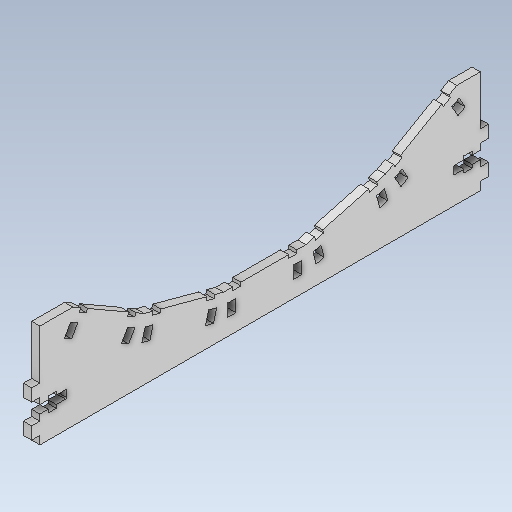
# Autodesk Inventor part: switchplate-support-04
Saved by Autodesk Inventor 2020.1 (Build 241239000, 239)
## iProperties
Created: 2019-06-27
Material: Acier, galvanisé
Document SubType Name: Modeling
Designer: Thibault
Density: 7.85 g/cm^3
Appearance: Anodisé - Bronze foncé subtil
Mass: 11.7255 g
Surface Area: 33.7109 cm^2
Volume: 1.4937 cm^3
Part Number: switchplate-support-04
sa_0: 0.400 nd
height_shift: 0,000 mm
base_height: 25,000 mm
switchplate_depth: 111,000 mm
Author: Thibault
Autodesk Inventor part; units mm, degrees
ref_plane "YZ Plane" through (0, 0, 0) normal (1, 0, 0) x (0, 1, 0)
ref_plane "XZ Plane" through (0, 0, 0) normal (0, 1, 0) x (-1, 0, 0)
ref_plane "XY Plane" through (0, 0, 0) normal (0, 0, 1) x (1, 0, 0)
sketch "Anchor (screw side)" plane through (0, 0, 0) normal (0, 0, 1) x (1, 0, 0)
  circle A0 centre (93.7814, 50.2592) radius 1
  line L0 (91.2814, 51.2592) -> (88.2814, 51.2592)
  line L1 (88.2814, 51.2592) -> (88.2814, 49.2592)
  line L2 (88.2814, 49.2592) -> (91.2814, 49.2592)
  line L3 (91.2814, 49.2592) -> (91.2814, 51.2592)
  line L4 (99.2814, 51.2592) -> (96.2814, 51.2592)
  line L5 (96.2814, 51.2592) -> (96.2814, 49.2592)
  line L6 (96.2814, 49.2592) -> (99.2814, 49.2592)
  line L7 (99.2814, 49.2592) -> (99.2814, 51.2592)
  line L8 (91.2814, 51.2592) -> (96.2814, 49.2592) construction
  line L9 (96.2814, 51.2592) -> (91.2814, 49.2592) construction
  line L10 (86.2814, 53.2592) -> (101.2814, 53.2592) construction
  line L11 (101.2814, 53.2592) -> (101.2814, 47.2592) construction
  line L12 (101.2814, 47.2592) -> (86.2814, 47.2592) construction
  line L13 (86.2814, 47.2592) -> (86.2814, 53.2592) construction
  point P0 (103.5798, 50.1132)
  dimension "d27_1" = 2
  dimension "d28_1" = 3
  dimension "d29" = 2
  dimension "d30" = 3
  dimension "d32" = 5
  dimension "d34" = 2
  dimension "d35" = 2
  dimension "d36" = 2
  dimension "d37" = 2
  measures "d27_1" diameter of A0
  measures "d28_1" distance of L2.end L1.end
  measures "d29" distance of L1.end L0.end
  measures "d30" distance of L6.end L5.end
  measures "d32" distance between parallel lines of L5 L3
  measures "d34" distance between parallel lines of L0 L10
  measures "d35" distance between parallel lines of L12 L2
  measures "d36" distance between parallel lines of L11 L7
  measures "d37" distance between parallel lines of L13 L1
sketch "Anchor (nut side)" plane through (0, 0, 0) normal (0, 0, 1) x (1, 0, 0)
  line L0 (10, 0) -> (8.5, 0)
  line L1 (8.5, 0) -> (8.5, -2)
  line L2 (8.5, -2) -> (9.3, -2)
  line L3 (9.3, -2) -> (9.3, -4)
  line L4 (5.7, -4) -> (5.7, -2)
  line L5 (5.7, -2) -> (6.5, -2)
  line L6 (6.5, -2) -> (6.5, 0)
  line L7 (6.5, 0) -> (5, 0)
  line L8 (2, 0) -> (2, 2)
  line L9 (2, 0) -> (3, 0) construction
  line L10 (2, 2) -> (5, 2)
  line L11 (5, 2) -> (5, 0)
  line L12 (5, 2) -> (7, 2) construction
  line L13 (10, 0) -> (10, 2)
  line L14 (10, 2) -> (13, 2)
  line L15 (13, 2) -> (13, 0)
  line L16 (0, 0) -> (2, 0)
  line L17 (13, 0) -> (15, 0)
  line L18 (5.7, -4) -> (6.5, -4)
  line L19 (9.3, -4) -> (8.5, -4)
  line L20 (6.5, -4) -> (6.5, -6.25)
  line L21 (8.5, -4) -> (8.5, -6.25)
  line L22 (6.75, -6.5) -> (7.5, -6.5)
  arc A0 (6.5, -6.25) -> (6.75, -6.5) centre (6.75, -6.25) ccw
  arc A1 (8.25, -6.5) -> (8.5, -6.25) centre (8.25, -6.25) ccw
  line L23 (7.5, -7.2938) -> (7.5, -4.9797)
  line L24 (7.5, -6.5) -> (8.25, -6.5)
  point P0 (9.1321, -0.6227)
  point P1 (6.5, -6.5)
  point P2 (8.5, -6.5)
  dimension "d3" = 2
  dimension "d7" = 5
  dimension "d10" = 1.5
  dimension "d11" = 2
  dimension "d12" = 0.8
  dimension "d13" = 2
  dimension "d14" = 0.8
  dimension "d15" = 2
  dimension "d18" = 2
  dimension "d19" = 0.8
  dimension "d20" = 0.8
  dimension "d21" = 2.5
  dimension "d22" = 2.5
  dimension "d23" = 2
  dimension "d38" = 2
  dimension "d39" = 0.25
  dimension "d118" = 2
  dimension "d120" = 3
  measures "d3" distance of point (0, 0) L8.start
  measures "d7" distance of L7.end L0.start
  measures "d10" distance of L0.start L0.end
  measures "d11" distance of L0.end L1.end
  measures "d12" distance of L1.end L2.end
  measures "d13" distance of L2.end L3.end
  measures "d14" distance of L4.end L5.end
  measures "d15" distance of L6.end L0.end
  measures "d18" distance of L15.end point (15, 0)
  measures "d19" distance of L4.start L18.end
  measures "d20" distance of L3.end L19.end
  measures "d21" distance of L18.end point (6.5, -6.5)
  measures "d22" distance of L19.end point (8.5, -6.5)
  measures "d23" distance of L18.end L19.end
  measures "d38" distance of the line from the sketch origin of L10
  measures "d39" radius of A0
  measures "d118" distance between parallel lines of L0 L14
  measures "d120" distance of L8.end L10.end
sketch "Anchor (to 2ndary key support)" plane through (0, 0, 0) normal (0, 0, 1) x (1, 0, 0)
  line L0 (12.7767, 14.8837) -> (14.7767, 14.8837)
  line L1 (14.7767, 14.8837) -> (14.7767, 11.8837)
  line L2 (14.7767, 11.8837) -> (12.7767, 11.8837)
  line L3 (12.7767, 11.8837) -> (12.7767, 14.8837)
  point P0 (14.0267, 11.8837)
  dimension "d40" = 2
  dimension "d41" = 3
  measures "d40" distance of L1.end L2.end
  measures "d41" distance of L0.end L1.end
sketch "Switch support" plane through (0, 0, 0) normal (0, 0, 1) x (1, 0, 0)
  line L0 (14.375, 16.4474) -> (15.075, 16.4474)
  line L1 (15.075, 16.4474) -> (15.075, 15.6474)
  line L2 (15.075, 15.6474) -> (17.075, 15.6474)
  line L3 (17.075, 15.6474) -> (17.075, 16.4474)
  line L4 (17.075, 16.4474) -> (22.875, 16.4474)
  line L5 (28.675, 16.4474) -> (28.675, 15.6474)
  line L6 (28.675, 15.6474) -> (30.675, 15.6474)
  line L7 (30.675, 15.6474) -> (30.675, 16.4474)
  line L8 (30.675, 16.4474) -> (31.375, 16.4474)
  line L9 (22.875, 19.1721) -> (22.875, 15.8971) construction
  line L10 (22.875, 16.4474) -> (28.675, 16.4474)
  line L11 (13.875, 13.6474) -> (15.875, 13.6474)
  line L12 (15.875, 13.6474) -> (15.875, 10.6474)
  line L13 (15.875, 10.6474) -> (13.875, 10.6474)
  line L14 (13.875, 10.6474) -> (13.875, 13.6474)
  line L15 (29.875, 13.6474) -> (31.875, 13.6474)
  line L16 (31.875, 13.6474) -> (31.875, 10.6474)
  line L17 (31.875, 10.6474) -> (29.875, 10.6474)
  line L18 (29.875, 10.6474) -> (29.875, 13.6474)
  point P0 (20.0288, 26.7181)
  dimension "d43" = 0.8
  dimension "d44" = 2
  dimension "d45" = 11.6
  dimension "d46" = 2
  dimension "d47" = 0.7
  dimension "d48" = 17
  dimension "d49" = 7
  dimension "d50" = 7
  dimension "d51" = 2
  measures "d43" distance of L1.start L1.end
  measures "d44" distance of L1.end L2.end
  measures "d45" distance of L5.start L3.end
  measures "d46" distance of L5.end L6.end
  measures "d47" distance of L7.end point (31.375, 16.447)
  measures "d48" distance of point (31.375, 16.447) point (14.375, 16.447)
  measures "d51" length of L2
sketch "Sketch1" plane through (0, 0, 0) normal (1, 0, 0) x (0, 1, 0)
  line L0 (0, -111) -> (25, -111)
  line L1 (0, 0) -> (0, -111)
  line L2 (25, 0) -> (0, 0)
  line L3 (25, -111) -> (25, -103.278)
  line L4 (24.4162, -11.0111) -> (25, -10)
  line L5 (28.2121, -16.9724) -> (22.1003, -16.9724)
  line L6 (24.25, -11.299) -> (25, -10)
  line L7 (15.75, -26.0215) -> (15, -27.3205)
  line L8 (21.9473, -35.6102) -> (15.8356, -35.6102)
  line L9 (14.6118, -28.7694) -> (15, -27.3205)
  line L10 (10.2118, -45.1901) -> (9.8236, -46.639)
  line L11 (19.8511, -55.1756) -> (13.7394, -55.1756)
  line L12 (9.8236, -48.139) -> (9.8236, -46.639)
  line L13 (9.8236, -65.139) -> (9.8236, -66.639)
  line L14 (22.0358, -74.7409) -> (15.9241, -74.7409)
  line L15 (10.2118, -68.0879) -> (9.8236, -66.639)
  line L16 (14.6118, -84.5087) -> (15, -85.9575)
  line L17 (28.3566, -93.3787) -> (22.2449, -93.3787)
  line L18 (15.75, -87.2566) -> (15, -85.9575)
  line L19 (24.25, -101.979) -> (25, -103.278)
  line L20 (25, 0) -> (25, -10)
  line L21 (14.6118, -28.7694) -> (14.4306, -29.4455)
  line L22 (14.4306, -29.4455) -> (13.6579, -29.2385)
  line L23 (13.6579, -29.2385) -> (13.1402, -31.1703)
  line L24 (13.1402, -31.1703) -> (13.913, -31.3774)
  line L25 (13.913, -31.3774) -> (12.4118, -36.9798)
  line L26 (10.9107, -42.5821) -> (10.1379, -42.3751)
  line L27 (10.1379, -42.3751) -> (9.6203, -44.3069)
  line L28 (9.6203, -44.3069) -> (10.393, -44.514)
  line L29 (10.393, -44.514) -> (10.2118, -45.1901)
  line L30 (15.0436, -37.685) -> (11.8802, -36.8373) construction
  line L31 (12.4118, -36.9798) -> (10.9107, -42.5821)
  line L32 (12.0366, -27.5617) -> (11.519, -29.4936)
  line L33 (11.519, -29.4936) -> (8.6212, -28.7171)
  line L34 (8.6212, -28.7171) -> (9.1388, -26.7853)
  line L35 (9.1388, -26.7853) -> (12.0366, -27.5617)
  line L36 (7.8955, -43.0166) -> (7.3778, -44.9484)
  line L37 (7.3778, -44.9484) -> (4.4801, -44.1719)
  line L38 (4.4801, -44.1719) -> (4.9977, -42.2401)
  line L39 (4.9977, -42.2401) -> (7.8955, -43.0166)
  line L40 (24.25, -11.299) -> (23.9, -11.9053)
  line L41 (23.9, -11.9053) -> (23.2072, -11.5053)
  line L42 (23.2072, -11.5053) -> (22.2072, -13.2373)
  line L43 (22.2072, -13.2373) -> (22.9, -13.6373)
  line L44 (22.9, -13.6373) -> (20, -18.6603)
  line L45 (17.1, -23.6832) -> (16.4072, -23.2832)
  line L46 (16.4072, -23.2832) -> (15.4072, -25.0153)
  line L47 (15.4072, -25.0153) -> (16.1, -25.4153)
  line L48 (16.1, -25.4153) -> (15.75, -26.0215)
  line L49 (22.3596, -20.0226) -> (19.5234, -18.3851) construction
  line L50 (20, -18.6603) -> (17.1, -23.6832)
  line L51 (22.0751, -9.466) -> (21.0751, -11.1981)
  line L52 (21.0751, -11.1981) -> (18.4771, -9.6981)
  line L53 (18.4771, -9.6981) -> (19.4771, -7.966)
  line L54 (19.4771, -7.966) -> (22.0751, -9.466)
  line L55 (14.0751, -23.3224) -> (13.0751, -25.0545)
  line L56 (13.0751, -25.0545) -> (10.4771, -23.5545)
  line L57 (10.4771, -23.5545) -> (11.4771, -21.8224)
  line L58 (11.4771, -21.8224) -> (14.0751, -23.3224)
  line L59 (9.8236, -48.139) -> (9.8236, -48.839)
  line L60 (9.8236, -48.839) -> (9.0236, -48.839)
  line L61 (9.0236, -48.839) -> (9.0236, -50.839)
  line L62 (9.0236, -50.839) -> (9.8236, -50.839)
  line L63 (9.8236, -50.839) -> (9.8236, -56.639)
  line L64 (9.8236, -62.439) -> (9.0236, -62.439)
  line L65 (9.0236, -62.439) -> (9.0236, -64.439)
  line L66 (9.0236, -64.439) -> (9.8236, -64.439)
  line L67 (9.8236, -64.439) -> (9.8236, -65.139)
  line L68 (12.5483, -56.639) -> (9.2733, -56.639) construction
  line L69 (9.8236, -56.639) -> (9.8236, -62.439)
  line L70 (7.0236, -47.639) -> (7.0236, -49.639)
  line L71 (7.0236, -49.639) -> (4.0236, -49.639)
  line L72 (4.0236, -49.639) -> (4.0236, -47.639)
  line L73 (4.0236, -47.639) -> (7.0236, -47.639)
  line L74 (7.0236, -63.639) -> (7.0236, -65.639)
  line L75 (7.0236, -65.639) -> (4.0236, -65.639)
  line L76 (4.0236, -65.639) -> (4.0236, -63.639)
  line L77 (4.0236, -63.639) -> (7.0236, -63.639)
  line L78 (10.2118, -68.0879) -> (10.393, -68.7641)
  line L79 (10.393, -68.7641) -> (9.6203, -68.9711)
  line L80 (9.6203, -68.9711) -> (10.1379, -70.903)
  line L81 (10.1379, -70.903) -> (10.9107, -70.6959)
  line L82 (10.9107, -70.6959) -> (12.4118, -76.2983)
  line L83 (13.913, -81.9007) -> (13.1402, -82.1077)
  line L84 (13.1402, -82.1077) -> (13.6579, -84.0396)
  line L85 (13.6579, -84.0396) -> (14.4306, -83.8325)
  line L86 (14.4306, -83.8325) -> (14.6118, -84.5087)
  line L87 (15.0436, -75.5931) -> (11.8802, -76.4407) construction
  line L88 (12.4118, -76.2983) -> (13.913, -81.9007)
  line L89 (7.3778, -68.3296) -> (7.8955, -70.2615)
  line L90 (7.8955, -70.2615) -> (4.9977, -71.038)
  line L91 (4.9977, -71.038) -> (4.4801, -69.1061)
  line L92 (4.4801, -69.1061) -> (7.3778, -68.3296)
  line L93 (11.519, -83.7845) -> (12.0366, -85.7163)
  line L94 (12.0366, -85.7163) -> (9.1388, -86.4928)
  line L95 (9.1388, -86.4928) -> (8.6212, -84.5609)
  line L96 (8.6212, -84.5609) -> (11.519, -83.7845)
  line L97 (15.75, -87.2566) -> (16.1, -87.8628)
  line L98 (16.1, -87.8628) -> (15.4072, -88.2628)
  line L99 (15.4072, -88.2628) -> (16.4072, -89.9948)
  line L100 (16.4072, -89.9948) -> (17.1, -89.5948)
  line L101 (17.1, -89.5948) -> (20, -94.6178)
  line L102 (22.9, -99.6407) -> (22.2072, -100.0407)
  line L103 (22.2072, -100.0407) -> (23.2072, -101.7728)
  line L104 (23.2072, -101.7728) -> (23.9, -101.3728)
  line L105 (23.9, -101.3728) -> (24.25, -101.979)
  line L106 (22.3596, -93.2555) -> (19.5234, -94.893) construction
  line L107 (20, -94.6178) -> (22.9, -99.6407)
  line L108 (13.0751, -88.2236) -> (14.0751, -89.9556)
  line L109 (14.0751, -89.9556) -> (11.4771, -91.4556)
  line L110 (11.4771, -91.4556) -> (10.4771, -89.7236)
  line L111 (10.4771, -89.7236) -> (13.0751, -88.2236)
  line L112 (21.0751, -102.08) -> (22.0751, -103.812)
  line L113 (22.0751, -103.812) -> (19.4771, -105.312)
  line L114 (19.4771, -105.312) -> (18.4771, -103.58)
  line L115 (18.4771, -103.58) -> (21.0751, -102.08)
  point P0 (24.25, -101.979)
  point P1 (15.75, -87.2566)
  point P2 (14.6118, -84.5087)
  point P3 (10.2118, -68.0879)
  point P4 (9.8236, -65.139)
  point P5 (9.8236, -48.139)
  point P6 (10.2118, -45.1901)
  point P7 (14.6118, -28.7694)
  point P8 (15.75, -26.0215)
  dimension "height" = 25
  dimension "d193" = 25
  dimension "k1_a" = 1.5
  dimension "k1_b" = 1.5
  dimension "k2_a" = 1.5
  dimension "k2_b" = 1.5
  dimension "k3_a" = 1.5
  dimension "k3_b" = 1.5
  dimension "k4_a" = 1.5
  dimension "k4_b" = 1.5
  dimension "k5_a" = 1.5
  dimension "k5_b" = 1.5
  dimension "d257" = 10
  dimension "k1_angle" = 120
  dimension "k2_angle" = 105
  dimension "k3_angle" = 90
  dimension "k4_angle" = 75
  dimension "k5_angle" = 60
  constraints: 42 end point, 7 horizontal, 4 vertical, 1 collinear, 1 vertical alignment, 19 other
  measures "height" distance of L2.start L1.start
  measures "d193" distance of L0.end L0.start
  measures "k1_a" distance of L4.end L6.start
  measures "k1_b" distance of L7.end L7.start
  measures "k2_a" distance of L9.start L7.end
  measures "k2_b" distance of L10.end L10.start
  measures "k3_a" distance of L12.start L10.end
  measures "k3_b" distance of L13.end L13.start
  measures "k4_a" distance of L15.start L13.end
  measures "k4_b" distance of L16.end L16.start
  measures "k5_a" distance of L18.start L16.end
  measures "k5_b" distance of L3.end L19.start
  measures "d257" distance of L2.start L4.end
  measures "k3_angle" angle to the sketch y axis of L11
extrude "Base" add sketch "Sketch1" along normal blind 2
sketch "Sketch2" plane through (0, 0, 0) normal (-1, 0, 0) x (0, 0, 1)
  line L0 (-109, 0) -> (-2, 0)
  line L1 (-179.6233, 19.237) -> (-179.6233, -29.346)
  line L2 (139.5944, 112.7524) -> (139.5944, -29.346)
  line L3 (139.5944, -29.346) -> (-179.6233, -29.346)
  line L4 (-111, 20) -> (-111, 0) construction
  line L5 (-109, 15) -> (-109, 103.8044)
  line L6 (-109, 103.8044) -> (-179.6233, 103.8044)
  line L7 (-179.6233, 103.8044) -> (-179.6233, 19.237)
  line L8 (-2, 15) -> (-2, 112.7524)
  line L9 (-2, 112.7524) -> (139.5944, 112.7524)
  line L10 (0, 0) -> (-111, 0) projected
  line L11 (-111, 0) -> (-111, 25) projected
  line L12 (0, 0) -> (-111, 0) projected
  line L13 (0, 25) -> (0, 0) projected
  line L14 (-109, 10) -> (-109, 8.5)
  line L15 (-109, 8.5) -> (-107, 8.5)
  line L16 (-107, 8.5) -> (-107, 9.3)
  line L17 (-107, 9.3) -> (-105, 9.3)
  line L18 (-105, 5.7) -> (-107, 5.7)
  line L19 (-107, 5.7) -> (-107, 6.5)
  line L20 (-107, 6.5) -> (-109, 6.5)
  line L21 (-109, 6.5) -> (-109, 5)
  line L22 (-109, 2) -> (-111, 2)
  line L23 (-109, 2) -> (-109, 3) construction
  line L24 (-111, 2) -> (-111, 5)
  line L25 (-111, 5) -> (-109, 5)
  line L26 (-111, 5) -> (-111, 7) construction
  line L27 (-109, 10) -> (-111, 10)
  line L28 (-111, 10) -> (-111, 13)
  line L29 (-111, 13) -> (-109, 13)
  line L30 (-109, 0) -> (-109, 2)
  line L31 (-109, 13) -> (-109, 15)
  line L32 (-105, 5.7) -> (-105, 6.5)
  line L33 (-105, 9.3) -> (-105, 8.5)
  line L34 (-105, 6.5) -> (-102.75, 6.5)
  line L35 (-105, 8.5) -> (-102.75, 8.5)
  line L36 (-102.5, 6.75) -> (-102.5, 7.5)
  arc A0 (-102.75, 6.5) -> (-102.5, 6.75) centre (-102.75, 6.75) ccw
  arc A1 (-102.5, 8.25) -> (-102.75, 8.5) centre (-102.75, 8.25) ccw
  line L37 (-101.7062, 7.5) -> (-104.0203, 7.5)
  line L38 (-102.5, 7.5) -> (-102.5, 8.25)
  line L39 (-2, 5) -> (-2, 6.5)
  line L40 (-2, 6.5) -> (-4, 6.5)
  line L41 (-4, 6.5) -> (-4, 5.7)
  line L42 (-4, 5.7) -> (-6, 5.7)
  line L43 (-6, 9.3) -> (-4, 9.3)
  line L44 (-4, 9.3) -> (-4, 8.5)
  line L45 (-4, 8.5) -> (-2, 8.5)
  line L46 (-2, 8.5) -> (-2, 10)
  line L47 (-2, 13) -> (0, 13)
  line L48 (-2, 13) -> (-2, 12) construction
  line L49 (0, 13) -> (0, 10)
  line L50 (0, 10) -> (-2, 10)
  line L51 (0, 10) -> (0, 8) construction
  line L52 (-2, 5) -> (0, 5)
  line L53 (0, 5) -> (0, 2)
  line L54 (0, 2) -> (-2, 2)
  line L55 (-2, 15) -> (-2, 13)
  line L56 (-2, 2) -> (-2, 0)
  line L57 (-6, 9.3) -> (-6, 8.5)
  line L58 (-6, 5.7) -> (-6, 6.5)
  line L59 (-6, 8.5) -> (-8.25, 8.5)
  line L60 (-6, 6.5) -> (-8.25, 6.5)
  line L61 (-8.5, 8.25) -> (-8.5, 7.5)
  arc A2 (-8.25, 8.5) -> (-8.5, 8.25) centre (-8.25, 8.25) ccw
  arc A3 (-8.5, 6.75) -> (-8.25, 6.5) centre (-8.25, 6.75) ccw
  line L62 (-9.2938, 7.5) -> (-6.9797, 7.5)
  line L63 (-8.5, 7.5) -> (-8.5, 6.75)
  point P0 (110, 20)
  point P1 (-110, 20)
  point P2 (-43.2578, 0)
  point P3 (-110, 14.3891)
  point P4 (0, 35.5246)
  point P5 (-110, 28.3499)
  point P6 (-111, 0)
  point P7 (-2, 0)
  point P8 (-109, 0)
  point P9 (-2, 0)
  constraints: 18 end point, 3 vertical, 2 horizontal, 2 parallel, 1 collinear, 1 perpendicular, 1 point on line, 10 other
extrude "Standard anchors" cut sketch "Sketch2" against normal through all
sketch "Esquisse7" plane through (0, 0, 0) normal (-1, 0, 0) x (0, 0, 1)
  line L0 (-104.5, 8.35) -> (-102.5, 8.35) construction
  line L1 (-106.5, 9.15) -> (-104.5, 9.15) construction
  line L2 (-104.5, 5.85) -> (-106.5, 5.85) construction
  line L3 (-102.5, 6.65) -> (-104.5, 6.65) construction
  line L4 (-109, 9.15) -> (-100.5, 9.15)
  line L5 (-109, 5.85) -> (-100.5, 5.85)
  line L6 (-109, 10) -> (-109, 8.35) construction
  line L7 (-109, 9.15) -> (-109, 5.85)
  arc A0 (-102.5, 6.65) -> (-102.5, 8.35) centre (-102.5, 7.5) ccw projected
  line L8 (-100.5, 5.85) -> (-100.5, 9.15)
  point P0 (1.5, 20)
  point P1 (108.5, 20)
  point P2 (108.5, 0)
  point P3 (1.5, 0)
  point P4 (-2, 10)
  point P5 (-2, 5)
  point P6 (7.6691, 10.85)
  point P7 (8.8147, 9.7576)
  point P8 (-111, 0)
  point P9 (-102.77, 8.35)
  point P10 (-100.7609, 7.9198)
  dimension "d203" = 2
  constraints: 8 end point, 2 collinear, 1 perpendicular, 1 vertical, 2 other
  measures "d203" distance from line of L8 A0.centre
extrude "No back screw hole" [suppressed]
sketch "Esquisse13" plane through (2, 0, 0) normal (1, 0, 0) x (0, 0, -1)
  line L0 (21.0345, 12.9637) -> (22.3023, 15.6826) projected
  line L1 (22.3023, 15.6826) -> (24.1149, 14.8374) projected
  line L2 (24.1149, 14.8374) -> (22.8471, 12.1185) projected
  line L3 (22.8471, 12.1185) -> (21.0345, 12.9637) projected
  point P0 (0, 0)
extrude "Hole fixup" [suppressed]
sketch "Esquisse8" plane through (0, 0, 0) normal (-1, 0, 0) x (0, 0, 1)
  line L0 (0, 0) -> (-111, 0) projected
  line L1 (0, 0) -> (-20.4545, 0)
  line L2 (0, 63.8513) -> (0, 0)
  line L3 (0, 25) -> (0, 0) projected
  line L4 (-25.4153, 63.8513) -> (0, 63.8513)
  line L5 (-25.4153, 63.8513) -> (-25.4153, 15)
  line L6 (-25.4153, 5) -> (-25.4153, 6.5)
  line L7 (-25.4153, 6.5) -> (-27.4153, 6.5)
  line L8 (-27.4153, 6.5) -> (-27.4153, 5.7)
  line L9 (-27.4153, 5.7) -> (-29.4153, 5.7)
  line L10 (-29.4153, 9.3) -> (-27.4153, 9.3)
  line L11 (-27.4153, 9.3) -> (-27.4153, 8.5)
  line L12 (-27.4153, 8.5) -> (-25.4153, 8.5)
  line L13 (-25.4153, 8.5) -> (-25.4153, 10)
  line L14 (-25.4153, 13) -> (-23.4153, 13)
  line L15 (-25.4153, 13) -> (-25.4153, 12) construction
  line L16 (-23.4153, 13) -> (-23.4153, 10)
  line L17 (-23.4153, 10) -> (-25.4153, 10)
  line L18 (-23.4153, 10) -> (-23.4153, 8) construction
  line L19 (-25.4153, 5) -> (-23.4153, 5)
  line L20 (-23.4153, 5) -> (-23.4153, 2)
  line L21 (-23.4153, 2) -> (-25.4153, 2)
  line L22 (-25.4153, 15) -> (-25.4153, 13)
  line L23 (-25.4153, 2) -> (-25.4153, 0)
  line L24 (-29.4153, 9.3) -> (-29.4153, 8.5)
  line L25 (-29.4153, 5.7) -> (-29.4153, 6.5)
  line L26 (-29.4153, 8.5) -> (-31.6653, 8.5)
  line L27 (-29.4153, 6.5) -> (-31.6653, 6.5)
  line L28 (-31.9153, 8.25) -> (-31.9153, 7.5)
  arc A0 (-31.6653, 8.5) -> (-31.9153, 8.25) centre (-31.6653, 8.25) ccw
  arc A1 (-31.9153, 6.75) -> (-31.6653, 6.5) centre (-31.6653, 6.75) ccw
  line L29 (-32.7091, 7.5) -> (-30.395, 7.5)
  line L30 (-31.9153, 7.5) -> (-31.9153, 6.75)
  point P0 (110, 0)
  point P1 (-109, 0)
  point P2 (0, 12.75)
  point P3 (0, 10.25)
  point P4 (0, 12)
  point P5 (-25.4153, 16.1)
  point P6 (-25.4153, 15)
  point P7 (-25.4153, 0)
  dimension "d232" = 20.4545
  constraints: 8 end point, 2 collinear, 2 horizontal, 2 vertical, 1 parallel, 1 point on line, 1 other
  measures "d232" distance of L0.start L1.end
extrude "Short plate" [suppressed]
derived "shared_parameters.ipt"
equation "\"depth_shift\" = 4"
equation "\"angle\" = 15deg"
equation "\"a_default\" = 1.5"
equation "\"b_default\" = 1.5"
